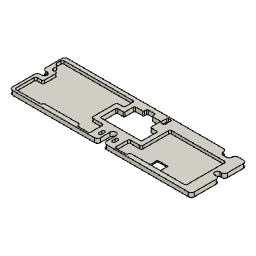
Frame Cover Plate Rev1.4 (Autodesk Fusion 360 design; units mm, degrees)
Autodesk Fusion 360 part; units mm, degrees
sketch "Sketch1" plane through (0, 0, 0) normal (0, 0, 1) x (1, 0, 0) in component "Cover"
  line L0 (69.75, 5.3) -> (63.75, 5.3)
  line L1 (47.25, 23.3) -> (47.25, 12.3)
  line L2 (69.75, 12.3) -> (69.75, 5.3)
  line L3 (74.75, 12.3) -> (69.75, 12.3)
  line L4 (63.75, 5.3) -> (63.75, 2.8)
  line L5 (52.25, 12.3) -> (52.25, 5.3)
  line L6 (63.75, 2.8) -> (58.25, 2.8)
  line L7 (47.25, 23.3) -> (74.75, 23.3)
  line L8 (47.25, 12.3) -> (52.25, 12.3)
  line L9 (58.25, 2.8) -> (58.25, 5.3)
  line L10 (74.75, 23.3) -> (74.75, 12.3)
  line L11 (52.25, 5.3) -> (58.25, 5.3)
  circle A0 centre (12.7254, 3.937) radius 0.45 construction
  line L12 (11.8504, 5.602) -> (11.8504, 7.352) construction
  line L13 (13.6004, 5.602) -> (11.8504, 5.602) construction
  line L14 (27.5938, 3.7375) -> (27.5938, 5.5875) construction
  line L15 (29.4438, 3.7375) -> (27.5938, 3.7375) construction
  circle A1 centre (28.5188, 4.6625) radius 0.5 construction
  circle A2 centre (26.0188, 4.6625) radius 0.925 construction
  circle A3 centre (12.7254, 6.477) radius 0.45 construction
  circle A4 centre (72.7364, 31.0857) radius 1.225 construction
  circle A5 centre (77.7364, 31.0857) radius 1.225 construction
  circle A6 centre (10.1854, 6.477) radius 0.875 construction
  circle A7 centre (10.1854, 3.937) radius 0.875 construction
  circle A8 centre (43.897, 31.0857) radius 1.225 construction
  circle A9 centre (48.897, 31.0857) radius 0.7 construction
  circle A10 centre (10.1854, 3.937) radius 0.45 construction
  circle A11 centre (48.897, 31.0857) radius 1.225 construction
  circle A12 centre (10.1854, 6.477) radius 0.45 construction
  circle A13 centre (77.7364, 31.0857) radius 0.7 construction
  line L16 (11.8504, 7.352) -> (13.6004, 7.352) construction
  circle A14 centre (35.3679, 34.0015) radius 0.875 construction
  circle A15 centre (8.4979, 19.224) radius 0.925 construction
  line L17 (13.6004, 7.352) -> (13.6004, 5.602) construction
  line L18 (7.5729, 15.149) -> (9.4229, 15.149) construction
  line L19 (37.0329, 34.8765) -> (38.7829, 34.8765) construction
  line L20 (9.4229, 15.149) -> (9.4229, 13.299) construction
  line L21 (9.4229, 13.299) -> (7.5729, 13.299) construction
  circle A16 centre (35.3679, 31.4615) radius 0.45 construction
  line L22 (28.3943, 33.0249) -> (26.6443, 33.0249) construction
  circle A17 centre (37.9079, 34.0015) radius 0.45 construction
  line L23 (7.5729, 13.299) -> (7.5729, 15.149) construction
  circle A18 centre (8.4979, 16.724) radius 0.925 construction
  circle A19 centre (43.897, 31.0857) radius 0.7 construction
  circle A20 centre (23.5188, 4.6625) radius 0.5 construction
  circle A21 centre (12.7254, 3.937) radius 0.875 construction
  circle A22 centre (8.4979, 14.224) radius 0.5 construction
  circle A23 centre (72.7364, 31.0857) radius 0.7 construction
  circle A24 centre (23.5188, 4.6625) radius 0.925 construction
  line L24 (38.7829, 34.8765) -> (38.7829, 33.1265) construction
  circle A25 centre (35.3679, 34.0015) radius 0.45 construction
  line L25 (29.4438, 5.5875) -> (29.4438, 3.7375) construction
  circle A26 centre (26.0188, 4.6625) radius 0.5 construction
  line L26 (37.0329, 33.1265) -> (37.0329, 34.8765) construction
  circle A27 centre (27.5193, 31.3599) radius 0.45 construction
  line L27 (38.7829, 33.1265) -> (37.0329, 33.1265) construction
  circle A28 centre (8.4979, 19.224) radius 0.5 construction
  circle A29 centre (35.3679, 31.4615) radius 0.875 construction
  circle A30 centre (24.9793, 33.8999) radius 0.875 construction
  circle A31 centre (8.4979, 21.724) radius 0.925 construction
  line L28 (27.5938, 5.5875) -> (29.4438, 5.5875) construction
  arc A32 (83.6167, 10.5889) -> (84.2667, 10.5889) centre (83.9417, 10.5889) ccw construction
  arc A33 (83.3167, 10.6139) -> (84.5667, 10.6139) centre (83.9417, 10.6139) ccw construction
  arc A34 (79.9067, 6.3739) -> (78.6567, 6.3739) centre (79.2817, 6.3739) ccw construction
  circle A35 centre (8.4979, 16.724) radius 0.5 construction
  line L29 (26.6443, 33.0249) -> (26.6443, 34.7749) construction
  circle A36 centre (112.7141, 21.9272) radius 0.925 construction
  circle A37 centre (24.9793, 31.3599) radius 0.875 construction
  line L30 (113.6391, 13.5022) -> (111.7891, 13.5022) construction
  circle A38 centre (81.6116, 12.4939) radius 0.35 construction
  line L31 (78.6567, 6.3739) -> (78.6567, 5.8739) construction
  line L32 (43.1948, 5.6637) -> (45.0448, 5.6637) construction
  circle A39 centre (37.9079, 31.4615) radius 0.45 construction
  circle A40 centre (36.6198, 4.7387) radius 0.925 construction
  circle A41 centre (27.5193, 31.3599) radius 0.875 construction
  circle A42 centre (39.1198, 4.7387) radius 0.925 construction
  line L33 (26.6443, 34.7749) -> (28.3943, 34.7749) construction
  line L34 (28.3943, 34.7749) -> (28.3943, 33.0249) construction
  line L35 (45.0448, 3.8137) -> (43.1948, 3.8137) construction
  circle A43 centre (36.6198, 4.7387) radius 0.5 construction
  line L36 (111.7891, 15.3522) -> (113.6391, 15.3522) construction
  circle A44 centre (27.5193, 33.8999) radius 0.45 construction
  line L37 (111.7891, 13.5022) -> (111.7891, 15.3522) construction
  circle A45 centre (24.9793, 33.8999) radius 0.45 construction
  arc A46 (78.6567, 5.8739) -> (79.9067, 5.8739) centre (79.2817, 5.8739) ccw construction
  circle A47 centre (112.7141, 16.9272) radius 0.5 construction
  arc A48 (78.9567, 5.8489) -> (79.6067, 5.8489) centre (79.2817, 5.8489) ccw construction
  circle A49 centre (112.7141, 14.4272) radius 0.5 construction
  circle A50 centre (81.6116, 4.4939) radius 0.35 construction
  circle A51 centre (112.7141, 21.9272) radius 0.5 construction
  circle A52 centre (24.9793, 31.3599) radius 0.45 construction
  line L38 (113.6391, 15.3522) -> (113.6391, 13.5022) construction
  line L39 (79.9067, 5.8739) -> (79.9067, 6.3739) construction
  circle A53 centre (112.7141, 16.9272) radius 0.925 construction
  circle A54 centre (112.7141, 19.4272) radius 0.925 construction
  circle A55 centre (112.7141, 19.4272) radius 0.5 construction
  circle A56 centre (81.6116, 4.4939) radius 0.475 construction
  circle A57 centre (39.1198, 4.7387) radius 0.5 construction
  circle A58 centre (44.1198, 4.7387) radius 0.5 construction
  circle A59 centre (8.4979, 21.724) radius 0.5 construction
  line L40 (43.1948, 3.8137) -> (43.1948, 5.6637) construction
  line L41 (45.0448, 5.6637) -> (45.0448, 3.8137) construction
  line L42 (79.9067, 10.6139) -> (79.9067, 11.1139) construction
  circle A60 centre (37.9079, 31.4615) radius 0.875 construction
  circle A61 centre (41.6198, 4.7387) radius 0.5 construction
  circle A62 centre (41.6198, 4.7387) radius 0.925 construction
  circle A63 centre (81.6116, 12.4939) radius 0.475 construction
  arc A64 (84.2667, 6.3989) -> (83.6167, 6.3989) centre (83.9417, 6.3989) ccw construction
  arc A65 (84.2667, 11.1389) -> (83.6167, 11.1389) centre (83.9417, 11.1389) ccw construction
  line L43 (84.2667, 10.5889) -> (84.2667, 11.1389) construction
  arc A66 (78.9567, 10.5889) -> (79.6067, 10.5889) centre (79.2817, 10.5889) ccw construction
  line L44 (78.6567, 11.1139) -> (78.6567, 10.6139) construction
  line L45 (84.5667, 5.8739) -> (84.5667, 6.3739) construction
  line L46 (79.6067, 5.8489) -> (79.6067, 6.3989) construction
  line L47 (83.3167, 6.3739) -> (83.3167, 5.8739) construction
  arc A67 (84.5667, 11.1139) -> (83.3167, 11.1139) centre (83.9417, 11.1139) ccw construction
  arc A68 (78.6567, 10.6139) -> (79.9067, 10.6139) centre (79.2817, 10.6139) ccw construction
  arc A69 (79.6067, 6.3989) -> (78.9567, 6.3989) centre (79.2817, 6.3989) ccw construction
  arc A70 (79.9067, 11.1139) -> (78.6567, 11.1139) centre (79.2817, 11.1139) ccw construction
  line L48 (78.9567, 11.1389) -> (78.9567, 10.5889) construction
  line L49 (83.3167, 11.1139) -> (83.3167, 10.6139) construction
  arc A71 (84.5667, 6.3739) -> (83.3167, 6.3739) centre (83.9417, 6.3739) ccw construction
  line L50 (78.9567, 6.3989) -> (78.9567, 5.8489) construction
  line L51 (79.6067, 10.5889) -> (79.6067, 11.1389) construction
  line L52 (84.2667, 5.8489) -> (84.2667, 6.3989) construction
  line L53 (83.6167, 6.3989) -> (83.6167, 5.8489) construction
  line L54 (83.6167, 11.1389) -> (83.6167, 10.5889) construction
  arc A72 (79.6067, 11.1389) -> (78.9567, 11.1389) centre (79.2817, 11.1389) ccw construction
  arc A73 (83.6167, 5.8489) -> (84.2667, 5.8489) centre (83.9417, 5.8489) ccw construction
  arc A74 (83.3167, 5.8739) -> (84.5667, 5.8739) centre (83.9417, 5.8739) ccw construction
  line L55 (84.5667, 10.6139) -> (84.5667, 11.1139) construction
  line L56 (61, 23.3) -> (61, 2.8) construction
  line L57 (0, 37) -> (122, 37)
  line L58 (122, 37) -> (122, 0)
  line L59 (122, 0) -> (0, 0)
  line L60 (0, 0) -> (0, 37)
  line L61 (61, 37) -> (61, 28.5) construction
  circle A75 centre (61, 28.5) radius 2
  line L62 (63, 28.5) -> (63, 37)
  line L63 (59, 28.5) -> (59, 37)
  circle A76 centre (3, 16.5) radius 1.75
  line L64 (3, 18.25) -> (0, 18.25)
  line L65 (3, 14.75) -> (0, 14.75)
  line L66 (119, 14.75) -> (122, 14.75)
  circle A77 centre (119, 16.5) radius 1.75
  line L67 (119, 18.25) -> (122, 18.25)
  line L68 (108.5, 0) -> (108.5, 4)
  line L69 (108.5, 4) -> (114.5, 4)
  line L70 (114.5, 4) -> (114.5, 0)
  line L71 (64.5, 32.55) -> (66.5, 32.55) construction
  line L72 (66.5, 32.55) -> (66.5, 30.55)
  line L73 (66.5, 30.55) -> (64.5, 30.55) construction
  line L74 (64.5, 30.55) -> (64.5, 32.55)
  circle A78 centre (65.5, 32.55) radius 1
  circle A79 centre (65.5, 30.55) radius 1
  circle A80 centre (56.5, 32.55) radius 1
  line L75 (57.5, 30.55) -> (57.5, 32.55)
  line L76 (55.5, 32.55) -> (55.5, 30.55)
  circle A81 centre (56.5, 30.55) radius 1
  line L77 (61, 28.5) -> (61, 23.3) construction
  point P0 (111.5, 4)
  dimension "d6" = 5.5
  dimension "d8" = 7
  dimension "d9" = 2.5
  dimension "d10" = 11
  dimension "d11" = 17.5
  dimension "d14" = 122
  dimension "d15" = 37
  dimension "d16" = 8.5
  dimension "d17" = 4
  dimension "d18" = 16.5
  dimension "d19" = 3
  dimension "d20" = 3.5
  dimension "d21" = 10.5
  dimension "d22" = 4
  dimension "d23" = 6
  dimension "d24" = 2
  dimension "d26" = 4.45
  dimension "d27" = 1.5
  dimension "d29" = 2
  dimension "d39" = 27.5
  dimension "d40" = 13.7
  constraint midpoint L7 L56.start
  constraint midpoint L6 L56.end
  constraint perpendicular L7 L56
  constraint equal L0 L11
  constraint perpendicular L3 L10
  constraint perpendicular L1 L8
  constraint perpendicular L5 L8
  constraint perpendicular L0 L2
  constraint perpendicular L5 L11
  constraint perpendicular L9 L11
  constraint perpendicular L0 L4
  constraint horizontal L6
  constraint equal L3 L8
  constraint equal L1 L10
  constraint horizontal L57
  constraint vertical L58
  constraint horizontal L59
  constraint vertical L60
  constraint coincident L59.end L60.start
  constraint midpoint L57 L61.start
  constraint perpendicular L57 L61
  constraint coincident L61.end A75.centre
  constraint coincident A75 L62.start
  constraint coincident L57 L62.end
  constraint perpendicular L57 L62
  constraint coincident A75 L63.start
  constraint coincident L57 L63.end
  constraint perpendicular L57 L63
  constraint tangent A75 L62
  constraint tangent A75 L63
  constraint coincident A76 L64.start
  constraint coincident L60 L64.end
  constraint perpendicular L60 L64
  constraint coincident A76 L65.start
  constraint coincident L60 L65.end
  constraint perpendicular L60 L65
  constraint tangent A76 L65
  constraint tangent A76 L64
  constraint symmetric L61 A76 A77
  constraint symmetric L61 L64.start L67.start
  constraint symmetric L61 L64.end L67.end
  constraint symmetric L61 L65.start L66.start
  constraint symmetric L61 L65.end L66.end
  constraint coincident L59 L68.start
  constraint perpendicular L59 L68
  constraint perpendicular L68 L69
  constraint coincident L59 L70.end
  constraint perpendicular L59 L70
  constraint midpoint L69 P0
  constraint horizontal L71
  constraint vertical L72
  constraint horizontal L73
  constraint vertical L74
  constraint midpoint L71 A78.centre
  constraint coincident L71.start A78
  constraint midpoint L73 A79.centre
  constraint coincident L73.end A79
  constraint symmetric L61 L71.start L75.end
  constraint symmetric L61 L71.end L76.start
  constraint symmetric L61 L72.end L76.end
  constraint symmetric L61 L73.end L75.start
  constraint symmetric L61 A78 A80
  constraint symmetric L61 A79 A81
  constraint perpendicular L1 L7
  constraint perpendicular L7 L10
  constraint equal L2 L5
  constraint parallel L61 L77
  measures "d6" distance of L4.end L6.end
  measures "d8" distance of L0.start L2.start
  measures "d9" distance of L0.end L4.end
  measures "d10" distance of L3.start L7.end
  measures "d11" distance of L2 L5
  measures "d14" distance of L57.start L57.end
  measures "d15" distance of L57.start L59.end
  measures "d16" distance of L61.start L61.end
  measures "d17" diameter of A75
  measures "d18" distance of L59 A76.centre
  measures "d19" distance of L60 A76.centre
  measures "d20" diameter of A76
  measures "d21" distance of L58 P0
  measures "d22" distance of L69.end L70.end
  measures "d23" distance of L68.end L69.end
  measures "d24" distance of L72.end L73.end
  measures "d26" distance of L57 L71.start
  measures "d27" distance of L62 L74
  measures "d29" distance of L71.end L72.end
  measures "d39" distance of L1.start L7.end
  measures "d40" distance of L7 L57
extrude "Extrude1" add sketch "Sketch1" against normal blind 3.2 contours L57 L58 L59 L60 A75 L62 L63 A76 L64 L65 L66 A77 L67 L68 L69 L70 in component "Cover"
sketch "Sketch2" plane through (0, 0, 0) normal (0, 0, 1) x (1, 0, 0) in component "Cover"
  arc A0 (64.5, 30.55) -> (66.5, 30.55) centre (65.5, 30.55) ccw
  line L0 (64.5, 30.55) -> (64.5, 32.55)
  arc A1 (66.5, 32.55) -> (64.5, 32.55) centre (65.5, 32.55) ccw
  arc A2 (57.5, 32.55) -> (55.5, 32.55) centre (56.5, 32.55) ccw
  line L1 (57.5, 32.55) -> (57.5, 30.55)
  arc A3 (55.5, 30.55) -> (57.5, 30.55) centre (56.5, 30.55) ccw
  line L2 (55.5, 30.55) -> (55.5, 32.55)
  line L3 (0, 18.25) -> (3, 18.25)
  line L4 (3, 14.75) -> (0, 14.75)
  arc A4 (64.5, 30.55) -> (66.5, 30.55) centre (65.5, 30.55) ccw
  line L5 (64.5, 30.55) -> (64.5, 32.55)
  arc A5 (66.5, 32.55) -> (64.5, 32.55) centre (65.5, 32.55) ccw
  line L6 (66.5, 32.55) -> (66.5, 30.55)
  line L7 (47.25, 12.3) -> (47.25, 23.3)
  line L8 (47.25, 23.3) -> (74.75, 23.3)
  line L9 (74.75, 23.3) -> (74.75, 12.3)
  line L10 (74.75, 12.3) -> (69.75, 12.3)
  line L11 (69.75, 12.3) -> (69.75, 5.3)
  line L12 (69.75, 5.3) -> (63.75, 5.3)
  line L13 (63.75, 5.3) -> (63.75, 2.8)
  line L14 (63.75, 2.8) -> (58.25, 2.8)
  line L15 (58.25, 2.8) -> (58.25, 5.3)
  line L16 (58.25, 5.3) -> (52.25, 5.3)
  line L17 (52.25, 5.3) -> (52.25, 12.3)
  line L18 (52.25, 12.3) -> (47.25, 12.3)
  arc A6 (57.5, 32.55) -> (55.5, 32.55) centre (56.5, 32.55) ccw
  line L19 (57.5, 32.55) -> (57.5, 30.55)
  arc A7 (55.5, 30.55) -> (57.5, 30.55) centre (56.5, 30.55) ccw
  line L20 (55.5, 30.55) -> (55.5, 32.55)
  line L21 (108.5, 0) -> (108.5, 4)
  line L22 (108.5, 4) -> (114.5, 4)
  line L23 (114.5, 4) -> (114.5, 0)
  line L24 (114.5, 0) -> (122, 0)
  line L25 (122, 0) -> (122, 14.75)
  line L26 (122, 14.75) -> (119, 14.75)
  arc A8 (119, 18.25) -> (119, 14.75) centre (119, 16.5) ccw
  line L27 (119, 18.25) -> (122, 18.25)
  line L28 (122, 18.25) -> (122, 37)
  line L29 (122, 37) -> (63, 37)
  line L30 (63, 37) -> (63, 28.5)
  arc A9 (59, 28.5) -> (63, 28.5) centre (61, 28.5) ccw
  line L31 (59, 28.5) -> (59, 37)
  line L32 (59, 37) -> (0, 37)
  line L33 (0, 37) -> (0, 18.25)
  line L34 (0, 18.25) -> (3, 18.25)
  arc A10 (3, 14.75) -> (3, 18.25) centre (3, 16.5) ccw
  line L35 (3, 14.75) -> (0, 14.75)
  line L36 (0, 14.75) -> (0, 0)
  line L37 (0, 0) -> (108.5, 0)
  line L38 (70.1, 1) -> (72.9, 1)
  line L39 (72.9, 1) -> (72.9, 6)
  line L40 (72.9, 6) -> (70.1, 6)
  line L41 (70.1, 6) -> (70.1, 1)
  line L42 (61, 2.8) -> (61, 0) construction
  line L43 (71.5, 1) -> (71.5, 0) construction
  line L44 (115.25, 34) -> (115.25, 7)
  line L45 (115.25, 7) -> (77.75, 7)
  line L46 (77.75, 7) -> (77.75, 26.3)
  line L47 (77.75, 26.3) -> (69.5, 26.3)
  line L48 (69.5, 26.3) -> (69.5, 36)
  line L49 (52.5, 36) -> (52.5, 26.3)
  line L50 (1.8, 35.4) -> (1.8, 21.25)
  line L51 (1.8, 21.25) -> (6.75, 21.25)
  line L52 (6.75, 21.25) -> (6.75, 11.75)
  line L53 (6.75, 11.75) -> (3, 11.75)
  line L54 (1, 2.5) -> (49.25, 2.5)
  line L55 (49.25, 2.5) -> (49.25, 9.3)
  line L56 (49.25, 9.3) -> (44.25, 9.3)
  line L57 (44.25, 9.3) -> (44.25, 26.3)
  line L58 (44.25, 26.3) -> (52.5, 26.3)
  line L59 (69.5, 36) -> (77.75, 36)
  line L60 (77.75, 36) -> (77.75, 34)
  line L61 (77.75, 34) -> (115.25, 34)
  line L62 (52.5, 36) -> (44.25, 36)
  line L63 (44.25, 36) -> (44.25, 34)
  line L64 (44.25, 34) -> (20, 34)
  line L65 (20, 34) -> (20, 35.4)
  line L66 (20, 35.4) -> (1.8, 35.4)
  line L67 (3, 11.75) -> (3, 7.5)
  line L68 (3, 7.5) -> (1, 7.5)
  line L69 (1, 7.5) -> (1, 2.5)
  dimension "d33" = 10.5
  dimension "d34" = 5
  dimension "d35" = 2.8
  dimension "d41" = 1
  dimension "d44" = 3.75
  dimension "d45" = 3
  dimension "d46" = 3
  dimension "d47" = 3
  dimension "d48" = 3
  dimension "d49" = 3
  dimension "d50" = 1
  dimension "d51" = 2.5
  dimension "d52" = 3
  dimension "d53" = 3
  dimension "d54" = 3
  dimension "d55" = 3
  dimension "d56" = 3
  dimension "d57" = 1
  dimension "d59" = 3
  dimension "d60" = 20
  dimension "d61" = 1.6
  dimension "d62" = 1.8
  dimension "d64" = 3.75
  dimension "d65" = 3
  dimension "d66" = 3
  dimension "d67" = 3
  dimension "d68" = 5
  dimension "d69" = 1
  constraint horizontal L38
  constraint vertical L39
  constraint horizontal L40
  constraint vertical L41
  constraint coincident L37 L42.end
  constraint perpendicular L37 L42
  constraint midpoint L38 L43.start
  constraint perpendicular L44 L45
  constraint perpendicular L45 L46
  constraint perpendicular L46 L47
  constraint perpendicular L8 L49
  constraint perpendicular L50 L51
  constraint perpendicular L51 L52
  constraint perpendicular L52 L53
  constraint perpendicular L54 L55
  constraint perpendicular L56 L57
  constraint coincident L49 L58.end
  constraint perpendicular L49 L58
  constraint coincident L37 L43.end
  constraint vertical L43
  constraint midpoint L14 L42.start
  constraint perpendicular L48 L59
  constraint perpendicular L59 L60
  constraint coincident L44 L61.end
  constraint perpendicular L44 L61
  constraint collinear L46 L60
  constraint perpendicular L49 L62
  constraint perpendicular L62 L63
  constraint coincident L50 L66.end
  constraint collinear L57 L63
  constraint perpendicular L63 L64
  constraint perpendicular L64 L65
  constraint perpendicular L65 L66
  constraint coincident L50.start L66
  constraint perpendicular L53 L67
  constraint perpendicular L67 L68
  constraint perpendicular L68 L69
  constraint coincident L54.start L69
  measures "d33" distance of L42.end L43.end
  measures "d34" distance of L38.end L39.end
  measures "d35" distance of L39.end L40.end
  measures "d41" distance of L37 L38
  measures "d44" distance of A8.centre L44
  measures "d45" distance of L22 L45
  measures "d46" distance of L9 L46
  measures "d47" distance of L8 L47
  measures "d48" distance of L6 L48
  measures "d49" distance of L29 L61
  measures "d50" distance of L29 L59
  measures "d51" distance of L37 L54
  measures "d52" distance of L17 L55
  measures "d53" distance of L18 L56
  measures "d54" distance of L7 L57
  measures "d55" distance of L8 L58
  measures "d56" distance of L2 L49
  measures "d57" distance of L32 L62
  measures "d59" distance of L32 L64
  measures "d60" distance of L33 L65.end
  measures "d61" distance of L32 L66
  measures "d62" distance of L33 L50
  measures "d64" distance of A10.centre L52
  measures "d65" distance of L3 L51
  measures "d66" distance of L4 L53
  measures "d67" distance of L36 L67
  measures "d68" distance of L54.start L68.end
  measures "d69" distance of L36 L69
extrude "Extrude2" cut sketch "Sketch2" along normal blind 2 from surface at -3.2 contours L38 L39 L40 L41 | L44 L45 L46 L47 L48 L59 L60 L61 | L49 L50 L51 L52 L53 L54 L55 L56 L57 L58 L62 L63 L64 L65 L66 L67 L68 L69 in component "Cover"
fillet "Fillet1" radius 2 14 edges at (59, 37, -1.6) (63, 37, -1.6) (0, 18.25, -1.6) (0, 14.75, -1.6) (0, 37, -1.6) (0, 0, -1.6) (122, 37, -1.6) (122, 18.25, -1.6) (122, 14.75, -1.6) (122, 0, -1.6) (114.5, 0, -1.6) (108.5, 0, -1.6) (108.5, 4, -1.6) (114.5, 4, -1.6) in component "Cover"
fillet "Fillet2" radius 0.6 16 edges at (52.25, 5.3, -1.6) (58.25, 2.8, -1.6) (63.75, 2.8, -1.6) (69.75, 5.3, -1.6) (74.75, 12.3, -1.6) (47.25, 12.3, -1.6) (47.25, 23.3, -1.6) (74.75, 23.3, -1.6) (52.25, 12.3, -1.6) (69.75, 12.3, -1.6) (58.25, 5.3, -1.6) (63.75, 5.3, -1.6) (70.1, 6, -2.2) (70.1, 1, -2.2) (72.9, 1, -2.2) (72.9, 6, -2.2) in component "Cover"
chamfer "Chamfer1" distance 0.4 angle 45 1 faces at (104.0631, 25.7682, 0) in component "Cover"
fillet "Fillet3" radius 1 26 edges at (69.5, 36, -2.2) (77.75, 36, -2.2) (77.75, 34, -2.2) (69.5, 26.3, -2.2) (115.25, 34, -2.2) (77.75, 26.3, -2.2) (77.75, 7, -2.2) (115.25, 7, -2.2) (44.25, 26.3, -2.2) (52.5, 26.3, -2.2) (52.5, 36, -2.2) (44.25, 36, -2.2) (44.25, 34, -2.2) (20, 34, -2.2) (20, 35.4, -2.2) (1.8, 35.4, -2.2) (1.8, 21.25, -2.2) (6.75, 21.25, -2.2) (6.75, 11.75, -2.2) (3, 11.75, -2.2) (3, 7.5, -2.2) (1, 7.5, -2.2) (1, 2.5, -2.2) (49.25, 2.5, -2.2) (49.25, 9.3, -2.2) (44.25, 9.3, -2.2) in component "Cover"
sketch "草图1" plane through (0, 0, 0) normal (0, 0, -1) x (1, 0, 0)
  arc A0 (57.9, 32.55) -> (55.1, 32.55) centre (56.5, 32.55) ccw
  line L0 (57.9, 32.55) -> (57.9, 30.55)
  arc A1 (55.1, 30.55) -> (57.9, 30.55) centre (56.5, 30.55) ccw
  line L1 (55.1, 30.55) -> (55.1, 32.55)
  arc A2 (64.1, 30.55) -> (66.9, 30.55) centre (65.5, 30.55) ccw
  line L2 (64.1, 30.55) -> (64.1, 32.55)
  arc A3 (66.9, 32.55) -> (64.1, 32.55) centre (65.5, 32.55) ccw
  line L3 (66.9, 32.55) -> (66.9, 30.55)
  arc A4 (64.35, 4.9) -> (64.15, 4.7) centre (64.35, 4.7) ccw
  line L4 (64.15, 4.7) -> (64.15, 3.4)
  arc A5 (63.15, 2.4) -> (64.15, 3.4) centre (63.15, 3.4) ccw
  line L5 (63.15, 2.4) -> (58.85, 2.4)
  arc A6 (57.85, 3.4) -> (58.85, 2.4) centre (58.85, 3.4) ccw
  line L6 (57.85, 3.4) -> (57.85, 4.7)
  arc A7 (57.85, 4.7) -> (57.65, 4.9) centre (57.65, 4.7) ccw
  line L7 (57.65, 4.9) -> (52.85, 4.9)
  arc A8 (51.85, 5.9) -> (52.85, 4.9) centre (52.85, 5.9) ccw
  line L8 (51.85, 5.9) -> (51.85, 11.7)
  arc A9 (51.85, 11.7) -> (51.65, 11.9) centre (51.65, 11.7) ccw
  line L9 (51.65, 11.9) -> (47.85, 11.9)
  arc A10 (46.85, 12.9) -> (47.85, 11.9) centre (47.85, 12.9) ccw
  line L10 (46.85, 12.9) -> (46.85, 22.7)
  arc A11 (47.85, 23.7) -> (46.85, 22.7) centre (47.85, 22.7) ccw
  line L11 (47.85, 23.7) -> (74.15, 23.7)
  arc A12 (75.15, 22.7) -> (74.15, 23.7) centre (74.15, 22.7) ccw
  line L12 (75.15, 22.7) -> (75.15, 12.9)
  arc A13 (74.15, 11.9) -> (75.15, 12.9) centre (74.15, 12.9) ccw
  line L13 (74.15, 11.9) -> (70.35, 11.9)
  arc A14 (70.35, 11.9) -> (70.15, 11.7) centre (70.35, 11.7) ccw
  line L14 (70.15, 11.7) -> (70.15, 5.9)
  arc A15 (69.15, 4.9) -> (70.15, 5.9) centre (69.15, 5.9) ccw
  line L15 (69.15, 4.9) -> (64.35, 4.9)
  arc A16 (106.5, 0.4) -> (108.1, 2) centre (106.5, 2) ccw
  arc A17 (110.5, 4.4) -> (108.1, 2) centre (110.5, 2) ccw
  line L16 (110.5, 4.4) -> (112.5, 4.4)
  arc A18 (114.9, 2) -> (112.5, 4.4) centre (112.5, 2) ccw
  arc A19 (114.9, 2) -> (116.5, 0.4) centre (116.5, 2) ccw
  line L17 (116.5, 0.4) -> (120, 0.4)
  arc A20 (120, 0.4) -> (121.6, 2) centre (120, 2) ccw
  line L18 (121.6, 2) -> (121.6, 12.75)
  arc A21 (121.6, 12.75) -> (120, 14.35) centre (120, 12.75) ccw
  line L19 (120, 14.35) -> (119, 14.35)
  arc A22 (119, 18.65) -> (119, 14.35) centre (119, 16.5) ccw
  line L20 (119, 18.65) -> (120, 18.65)
  arc A23 (120, 18.65) -> (121.6, 20.25) centre (120, 20.25) ccw
  line L21 (121.6, 20.25) -> (121.6, 35)
  arc A24 (121.6, 35) -> (120, 36.6) centre (120, 35) ccw
  line L22 (120, 36.6) -> (65, 36.6)
  arc A25 (65, 36.6) -> (63.4, 35) centre (65, 35) ccw
  line L23 (63.4, 35) -> (63.4, 28.5)
  arc A26 (58.6, 28.5) -> (63.4, 28.5) centre (61, 28.5) ccw
  line L24 (58.6, 28.5) -> (58.6, 35)
  arc A27 (58.6, 35) -> (57, 36.6) centre (57, 35) ccw
  line L25 (57, 36.6) -> (2, 36.6)
  arc A28 (2, 36.6) -> (0.4, 35) centre (2, 35) ccw
  line L26 (0.4, 35) -> (0.4, 20.25)
  arc A29 (0.4, 20.25) -> (2, 18.65) centre (2, 20.25) ccw
  line L27 (2, 18.65) -> (3, 18.65)
  arc A30 (3, 14.35) -> (3, 18.65) centre (3, 16.5) ccw
  line L28 (3, 14.35) -> (2, 14.35)
  arc A31 (2, 14.35) -> (0.4, 12.75) centre (2, 12.75) ccw
  line L29 (0.4, 12.75) -> (0.4, 2)
  arc A32 (0.4, 2) -> (2, 0.4) centre (2, 2) ccw
  line L30 (2, 0.4) -> (106.5, 0.4)
  line L31 (120, 37) -> (65, 37)
  line L32 (122, 20.25) -> (122, 35)
  line L33 (92.8, 37) -> (92.8, 30.5) construction
  line L34 (92.8, 30.5) -> (122, 30.5) construction
  line L35 (96.3, 27) -> (89.3, 27)
  line L36 (89.3, 27) -> (89.3, 34)
  line L37 (89.3, 34) -> (96.3, 34)
  line L38 (96.3, 34) -> (96.3, 27)
  line L39 (96.3, 27) -> (89.3, 34) construction
  line L40 (89.3, 27) -> (96.3, 34) construction
  point P0 (92.8, 30.5)
  dimension "d78" = 6.5
  dimension "d79" = 29.2
  dimension "d80" = 7
  dimension "d81" = 7
  constraint coincident L31 L33.start
  constraint coincident L32 L34.end
  constraint perpendicular L32 L34
  constraint horizontal L35
  constraint perpendicular L35 L36
  constraint parallel L35 L37
  constraint parallel L36 L38
  constraint coincident L39 P0
  constraint coincident L40 P0
  constraint coincident P0 L33.end
  measures "d78" distance of L33.start P0
  measures "d79" distance of P0 L34.end
  measures "d80" distance of L36.end L37.end
  measures "d81" distance of L35.end L36.end
extrude "拉伸3" cut sketch "草图1" against normal blind 18 contours L35 L36 L37 L38 sketch seen with x (1, 0, 0) y (0, -1, 0) z (0, 0, -1) at (0, 0, 0) in component "Cover"
chamfer "倒角2" distance 0.4 angle 45 4 edges at (92.8, 34, 0) (89.3, 30.5, 0) (96.3, 30.5, 0) (92.8, 27, 0) in component "Cover"
component "Cover" placed x (1, 0, 0) y (0, -1, 0) z (0, 0, -1) at (0, 0, 0)
equation "d44 = 1.75 mm + 2 mm"
